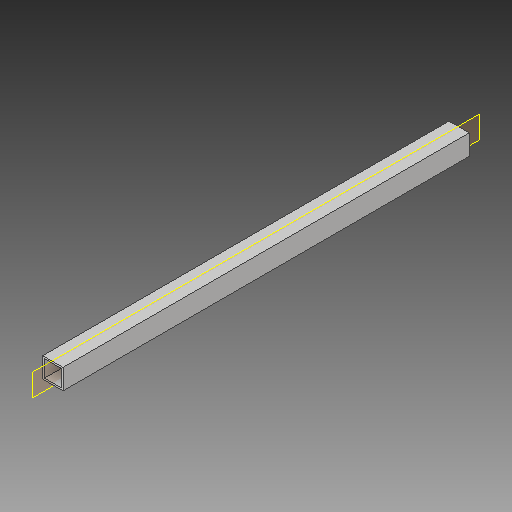
# Autodesk Inventor part: 1_5inSquareArmTube
Saved by Autodesk Inventor 2019 (Build 230136000, 136)
## iProperties
Created: 2018-02-07
Part Number: 1_5inSquareArmTube
Material: Generic
Document SubType Name: Modeling
Designer: steele
Density: 1 g/cm^3
Appearance: Default
Author: steele
Autodesk Inventor part; units mm, degrees
ref_plane "XZ Plane" through (0, 0, 0) normal (0, 1, 0) x (-1, 0, 0)
ref_plane "XY Plane" through (0, 0, 0) normal (0, 0, 1) x (1, 0, 0)
sketch "Sketch1" plane through (0, 0, 0) normal (0, 0, 1) x (1, 0, 0)
  line L0 (-19.05, -19.05) -> (19.05, -19.05)
  line L1 (19.05, -19.05) -> (19.05, 19.05)
  line L2 (19.05, 19.05) -> (-19.05, 19.05)
  line L3 (-19.05, 19.05) -> (-19.05, -19.05)
  line L4 (-19.05, -19.05) -> (19.05, 19.05) construction
  line L5 (19.05, -19.05) -> (-19.05, 19.05) construction
  line L6 (-15.875, -15.875) -> (15.875, -15.875)
  line L7 (15.875, -15.875) -> (15.875, 15.875)
  line L8 (15.875, 15.875) -> (-15.875, 15.875)
  line L9 (-15.875, 15.875) -> (-15.875, -15.875)
  line L10 (-15.875, -15.875) -> (15.875, 15.875) construction
  line L11 (15.875, -15.875) -> (-15.875, 15.875) construction
  point P0 (0, 0)
  dimension "d0" = 38.1
  dimension "d1" = 3.175
  constraints: 24 end point, 4 midpoint, 4 parallel, 4 perpendicular, 2 horizontal
  measures "d0" distance of L0.start L0.end
  measures "d1" distance between parallel lines of L6 L0
extrude "Extrusion1" add sketch "Sketch1" against normal blind 762
body "Solid1"
